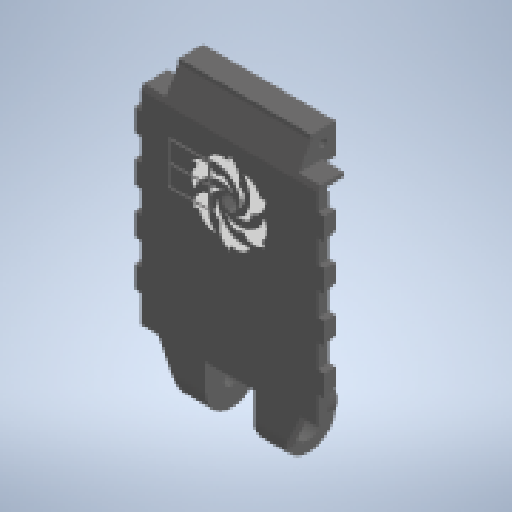
# Autodesk Inventor part: protector
Saved by Autodesk Inventor 2026.1 (Build 301233020, 233B)
## iProperties
Created: 2026-01-21
Part Number: protector
Material: 一般
Document SubType Name: Modeling
Designer: hibik
Density: 1 g/cm^3
Appearance: 既定
Author: hibik
Autodesk Inventor part; units mm, degrees
ref_plane "YZ Plane" through (0, 0, 0) normal (1, 0, 0) x (0, 1, 0)
ref_plane "XZ Plane" through (0, 0, 0) normal (0, 1, 0) x (-1, 0, 0)
ref_plane "XY Plane" through (0, 0, 0) normal (0, 0, 1) x (1, 0, 0)
sketch "スケッチ1" plane through (0, 0, 0) normal (0, 0, 1) x (1, 0, 0)
  line L0 (-20, 22.5) -> (20, 22.5)
  line L1 (20, 22.5) -> (20, -22.5)
  line L2 (20, -22.5) -> (-20, -22.5)
  line L3 (-20, -22.5) -> (-20, 22.5)
  line L4 (-20, 22.5) -> (20, -22.5) construction
  line L5 (20, 22.5) -> (-20, -22.5) construction
  circle A0 centre (-17, 19.5) radius 3
  circle A1 centre (17, -19.5) radius 3
  point P0 (0, 0)
  point P1 (-20, 19.5)
  point P2 (17, -22.5)
  point P3 (20, -19.5)
  point P4 (-17, 22.5)
  dimension "d0" = 40
  dimension "d1" = 45
  dimension "d2" = 6
  constraints: 12 end point, 4 tangent, 2 centre point, 2 midpoint, 2 parallel, 1 equal radius, 1 horizontal, 1 perpendicular
  measures "d0" distance of L0.start L0.end
  measures "d1" distance of L2.end L0.start
  measures "d2" diameter of A0
extrude "押し出し1" add sketch "スケッチ1" along normal blind 0.5 contours L0 L1 A1 L2 L3 A0 | A0 | A1
sketch "スケッチ2" plane through (0, 0, 0) normal (0, 0, -1) x (-1, 0, 0)
  circle A0 centre (17, 19.5) radius 3
  circle A1 centre (-17, -19.5) radius 3
  arc A2 (20, 19.5) -> (17, 22.5) centre (17, 19.5) ccw projected
  arc A3 (-20, -19.5) -> (-17, -22.5) centre (-17, -19.5) ccw projected
  point P0 (0, 0)
  constraints: 4 concentric, 2 centre point
extrude "押し出し2" add sketch "スケッチ2" along normal blind 2
sketch "スケッチ3" plane through (17, -19.5, -2) normal (0, 0, -1) x (-1, 0, 0)
  circle A0 centre (34, 39) radius 1.25
  circle A1 centre (0, 0) radius 1.25
  circle A2 centre (34, 39) radius 3 construction
  circle A3 centre (0, 0) radius 3 construction
  point P0 (17, 19.5)
  dimension "d7" = 2.5
  constraints: 2 centre point, 2 concentric, 1 equal radius
  measures "d7" diameter of A0
extrude "押し出し3" cut sketch "スケッチ3" against normal through all
sketch "スケッチ4" plane through (0, 0, 0.5) normal (0, 0, 1) x (1, 0, 0)
  circle A0 centre (105.92, 111.13) radius 1.6667 projected
  line L0 (-14, 17.5) -> (-4, 17.5)
  line L1 (-4, 17.5) -> (-4, 7.5)
  line L2 (-4, 7.5) -> (-14, 7.5)
  line L3 (-14, 7.5) -> (-14, 17.5)
  line L4 (20, 22.5) -> (-17, 22.5) projected
  line L5 (-20, 19.5) -> (-20, -22.5) projected
  point P0 (0, 0)
  dimension "d10" = 5
  dimension "d11" = 6
  dimension "d12" = 10
  dimension "d13" = 10
  constraints: 8 end point, 2 parallel, 1 horizontal, 1 perpendicular
  measures "d10" distance between parallel lines of L4 L0
  measures "d11" distance between parallel lines of L5 L3
  measures "d12" distance of L0.start L0.end
  measures "d13" distance of L2.end L0.start
extrude "押し出し4" cut sketch "スケッチ4" against normal through all
sketch "スケッチ5" plane through (0, 0, 0.5) normal (0, 0, 1) x (1, 0, 0)
  line L0 (-20, 29.5) -> (20, 29.5)
  line L1 (20, 29.5) -> (20, -22.5)
  line L2 (20, -22.5) -> (-20, -22.5)
  line L3 (-20, -22.5) -> (-20, 29.5)
  line L4 (20, -19.5) -> (20, 22.5) projected
  line L5 (-20, 19.5) -> (-20, -22.5) projected
  line L6 (-20, -22.5) -> (17, -22.5) projected
  line L7 (20, 22.5) -> (-17, 22.5) projected
  line L8 (-14, 17.5) -> (-4, 17.5) projected
  line L9 (-4, 17.5) -> (-4, 7.5) projected
  line L10 (-4, 7.5) -> (-14, 7.5) projected
  line L11 (-14, 7.5) -> (-14, 17.5) projected
  circle A0 centre (0, 11.28) radius 1.6667 projected
  point P0 (0, 0)
  dimension "d16" = 7
  constraints: 8 end point, 3 point on line, 2 parallel, 1 horizontal, 1 perpendicular
  measures "d16" distance between parallel lines of L7 L0
extrude "押し出し5" add sketch "スケッチ5" along normal blind 2
sketch "スケッチ6" plane through (20, -19.5, 0) normal (1, 0, 0) x (0, 0, -1)
  circle A0 centre (3.5, -9) radius 6
  line L0 (-2.5, -3) -> (-2.5, 49) projected
  line L1 (-0.5, -3) -> (-2.5, -3) projected
  line L2 (-0.5, -3) -> (3.5, -3)
  line L3 (-2.5, -3) -> (-2.5, -9)
  point P0 (0, 19.5)
  dimension "d19" = 12
  constraints: 4 end point, 4 tangent, 2 point on circle, 1 centre point
  measures "d19" diameter of A0
extrude "押し出し6" add sketch "スケッチ6" against normal up to surface (40 mm away)
sketch "スケッチ7" plane through (0, 0, 0.5) normal (0, 0, -1) x (-1, 0, 0)
  line L0 (20, 29.5) -> (20, 19.5) projected
  line L1 (-20, 29.5) -> (20, 29.5)
  line L2 (20, 29.5) -> (20, 23.5)
  line L3 (20, 23.5) -> (-20, 23.5)
  line L4 (-20, 23.5) -> (-20, 29.5)
  line L5 (-10, 29.5) -> (10, 29.5)
  line L6 (10, 29.5) -> (10, 23.5)
  line L7 (10, 23.5) -> (-10, 23.5)
  line L8 (-10, 23.5) -> (-10, 29.5)
  line L9 (-20, 22.5) -> (17, 22.5) projected
  line L10 (-11, 29.5) -> (-11, 23.5)
  line L11 (11, 23.5) -> (11, 29.5)
  line L12 (0, 29.5) -> (0, 23.5)
  point P0 (0, 0)
  dimension "d22" = 1
  dimension "d23" = 20
  dimension "d24" = 22
  constraints: 22 end point, 7 point on line, 4 parallel, 4 perpendicular, 3 midpoint, 2 horizontal, 1 other
  measures "d22" distance between parallel lines of L3 L9
  measures "d23" distance between parallel lines of L6 L8
  measures "d24" distance between parallel lines of L10 L11
extrude "押し出し7" cut sketch "スケッチ7" against normal through all contours L0 L3 L11 L1 | L10 L3 L4 L1
extrude "押し出し8" add sketch "スケッチ7" along normal blind 7 contours L11 L3 L6 L1 | L8 L3 L10 L1
extrude "押し出し9" add sketch "スケッチ7" along normal blind 3.5 contours L6 L3 L12 L1 | L12 L3 L8 L1
sketch "スケッチ8" plane through (11, 23.5, 2.5) normal (1, 0, 0) x (0, 0, -1)
  line L0 (0, 0) -> (3.5, 6)
  line L1 (3.5, 6) -> (5.5, 6)
  line L2 (5.5, 6) -> (2, 0)
  line L3 (0, 0) -> (0, 6) projected
  line L4 (0, 6) -> (9, 6) projected
  point P0 (2.5, -23.5)
  constraints: 6 end point, 1 horizontal, 1 parallel
extrude "押し出し10" cut sketch "スケッチ8" against normal through all
sketch "スケッチ9" plane through (0, 0, -6.5) normal (0, 0, -1) x (-1, 0, 0)
  line L0 (-10, 29.5) -> (-11, 29.5) projected
  line L1 (10, 23.5) -> (11, 23.5) projected
  line L2 (-11, 29.5) -> (11, 29.5)
  line L3 (11, 29.5) -> (11, 23.5)
  line L4 (11, 23.5) -> (-11, 23.5)
  line L5 (-11, 23.5) -> (-11, 29.5)
  point P0 (0, 0)
  constraints: 8 end point, 2 parallel, 1 horizontal, 1 perpendicular
extrude "押し出し11" add sketch "スケッチ9" against normal blind 1
sketch "スケッチ10" plane through (-11, 29.5, -6.5) normal (0, 1, 0) x (1, 0, 0)
  line L0 (0, 0) -> (22, 0) projected
  line L1 (0, -5.5) -> (0, 0) projected
  line L2 (0, -5.5) -> (22, -5.5) projected
  line L3 (22, -5.5) -> (22, 0) projected
  line L4 (21, -1) -> (1, -1) projected
  line L5 (21, -3.5) -> (21, -1) projected
  line L6 (1, -3.5) -> (21, -3.5) projected
  line L7 (1, -3.5) -> (1, -1) projected
  point P0 (11, -6.5)
extrude "押し出し12" add sketch "スケッチ10" along normal blind 1 contours L0 L3 L2 L1 | L5 L6 L7 L4
sketch "スケッチ11" plane through (-20, 23.5, 2.5) normal (0, 1, 0) x (1, 0, 0)
  line L0 (9, 0) -> (9, 3.5) projected
  line L1 (31, 3.5) -> (31, 0) projected
  line L2 (31, 3.5) -> (31, 9) projected
  line L3 (9, 9) -> (9, 3.5) projected
  line L4 (0, 0) -> (0, 2) projected
  line L5 (0, 0) -> (9, 0)
  line L6 (9, 0) -> (9, 6)
  line L7 (9, 6) -> (0, 6)
  line L8 (0, 6) -> (0, 0)
  line L9 (40, 0) -> (31, 0)
  line L10 (31, 0) -> (31, 6)
  line L11 (31, 6) -> (40, 6)
  line L12 (40, 6) -> (40, 0)
  point P0 (20, 2.5)
  dimension "d41" = 6
  constraints: 16 end point, 4 parallel, 4 point on line, 2 horizontal, 2 perpendicular
  measures "d41" distance of L7.end L4.start
extrude "押し出し13" add sketch "スケッチ11" along normal blind 1
sketch "スケッチ12" plane through (-20, -22.5, 0) normal (-1, 0, 0) x (0, 0, 1)
  line L0 (1.9167, 47) -> (2.5, 46) projected
  line L1 (2.5, 46) -> (2.5, 47) projected
  line L2 (1.9167, 47) -> (2.5, 47) projected
  point P0 (0, 22.5)
extrude "押し出し14" cut sketch "スケッチ12" against normal through all
sketch "スケッチ13" plane through (0, 0, 0) normal (1, 0, 0) x (0, 1, 0)
  line L0 (24.5, 1.9167) -> (23.5, 2.5) projected
  line L1 (23.5, 2.5) -> (-28.5, 2.5) projected
  arc A0 (-28.5, 2.5) -> (-22.5, -3.5) centre (-28.5, -3.5) ccw projected
  line L2 (-22.5, -3.5) -> (-22.5, 0.5) projected
  line L3 (-22.5, 0.5) -> (-19.5, 0.5) projected
  line L4 (-19.5, 0) -> (-19.5, 0.5) projected
  line L5 (-19.5, 0) -> (22.5, 0) projected
  line L6 (22.5, 0) -> (22.5, 0.5) projected
  line L7 (22.5, 0.5) -> (23.5, 0.5) projected
  line L8 (23.5, 0.5) -> (23.5, -3.5) projected
  line L9 (23.5, -3.5) -> (24.5, -3.5) projected
  line L10 (24.5, 1.9167) -> (24.5, -3.5) projected
  line L11 (-22.5, 0.5) -> (-22.5, 2.5)
  point P0 (0, 0)
  constraints: 2 end point, 1 perpendicular, 1 point on line
extrude "押し出し15" cut sketch "スケッチ13" along normal mid plane 11 contours L11 L2 A0 L1
sketch "スケッチ14" plane through (20, -19.5, 0) normal (1, 0, 0) x (0, 0, -1)
  line L0 (-1.9167, 44) -> (-2.5, 43) projected
  line L1 (-2.5, 43) -> (-2.5, -9) projected
  arc A0 (-2.5, -9) -> (3.5, -3) centre (3.5, -9) ccw projected
  line L2 (3.5, -3) -> (-0.5, -3) projected
  line L3 (-0.5, -3) -> (-0.5, 0) projected
  line L4 (0, 0) -> (-0.5, 0) projected
  line L5 (0, 0) -> (0, 42) projected
  line L6 (0, 42) -> (-0.5, 42) projected
  line L7 (-0.5, 42) -> (-0.5, 43) projected
  line L8 (-0.5, 43) -> (3.5, 43) projected
  line L9 (3.5, 43) -> (3.5, 44) projected
  line L10 (-1.9167, 44) -> (3.5, 44) projected
  line L11 (-0.5, -3) -> (-2.5, -3)
  point P0 (0, 19.5)
  constraints: 2 end point, 1 perpendicular, 1 point on line
extrude "押し出し16" cut sketch "スケッチ14" against normal blind 8 contours L11 L2 A0 L1
chamfer "面取り3" distance 4 distance2 9 2 edges at (12, -22.5, 1.5) (12, -22.5, 0.25) measured on face at (12.5, -22.5, 0.25) measured on face at (12.5, -22.5, 1.5)
sketch "スケッチ15" plane through (12, -19.5, 0) normal (1, 0, 0) x (0, 0, -1)
  line L0 (-1.6962, -12) -> (0, -12) projected
  arc A0 (-1.6962, -12) -> (3.5, -3) centre (3.5, -9) ccw projected
  line L1 (0, -3) -> (3.5, -3) projected
  line L2 (0, -3) -> (0, -12) projected
  circle A1 centre (3.5, -9) radius 1.75
  point P0 (0, 19.5)
  dimension "d56" = 3.5
  constraints: 1 centre point, 1 coincident
  measures "d56" diameter of A1
extrude "押し出し17" cut sketch "スケッチ15" against normal through all contours A1
mirror "ミラー1" about plane through (0, 0, 0) normal (1, 0, 0) of "押し出し16", "面取り3"
sketch "スケッチ16" plane through (12, -19.5, 0) normal (1, 0, 0) x (0, 0, -1)
  circle A0 centre (3.5, -9) radius 1.75 projected
  circle A1 centre (3.5, -9) radius 3.5
  point P0 (0, 19.5)
  dimension "d59" = 7
  constraints: 1 centre point, 1 coincident
  measures "d59" diameter of A1
extrude "押し出し18" cut sketch "スケッチ16" against normal blind 3
sketch "スケッチ17" plane through (-12, -31.5, 0) normal (-1, 0, 0) x (0, 0, 1)
  circle A0 centre (-3.5, 3) radius 1.75 projected
  arc A1 (-3.5, 9) -> (2.5, 3) centre (-3.5, 3) ccw projected
  line L0 (-3.5, -1.0415) -> (-7, 0.9793)
  line L1 (-7, 0.9793) -> (-7, 5.0207)
  line L2 (-7, 5.0207) -> (-3.5, 7.0415)
  line L3 (-3.5, 7.0415) -> (0, 5.0207)
  line L4 (0, 5.0207) -> (0, 0.9793)
  line L5 (0, 0.9793) -> (-3.5, -1.0415)
  point P0 (0, 31.5)
  dimension "d62" = 7
  constraints: 12 end point, 1 coincident, 1 vertical, 13 other
  measures "d62" distance between parallel lines of L4 L1
extrude "押し出し19" cut sketch "スケッチ17" against normal blind 3
sketch "スケッチ18" plane through (0, 0, 0) normal (0, 0, -1) x (-1, 0, 0)
  line L0 (4, 12.75) -> (13.5, 12.75)
  line L1 (13.5, 12.75) -> (13.5, 17)
  line L2 (13.5, 17) -> (4, 17)
  line L3 (4, 17) -> (4, 12.75)
  line L4 (4, 12.25) -> (13.5, 12.25)
  line L5 (13.5, 12.25) -> (13.5, 8)
  line L6 (13.5, 8) -> (4, 8)
  line L7 (4, 8) -> (4, 12.25)
  line L8 (4, 7.5) -> (4, 17.5) projected
  line L9 (14, 17.5) -> (14, 7.5) projected
  line L10 (4, 17.5) -> (14, 17.5) projected
  line L11 (14, 7.5) -> (4, 7.5) projected
  point P0 (0, 0)
  dimension "d65" = 0.5
  dimension "d66" = 0.5
  dimension "d67" = 0.5
  dimension "d68" = 0.5
  constraints: 16 end point, 4 parallel, 3 collinear, 2 horizontal, 2 perpendicular, 1 point on line
  measures "d65" distance between parallel lines of L9 L5
  measures "d66" distance between parallel lines of L0 L4
  measures "d67" distance between parallel lines of L10 L2
  measures "d68" distance between parallel lines of L11 L6
extrude "押し出し20" add sketch "スケッチ18" against normal blind 1 contours L3 L2 L1 L0 | L4 L5 L6 L7
sketch "スケッチ19" plane through (0, 0, 1) normal (0, 0, 1) x (1, 0, 0)
  line L0 (-4, 17) -> (-13.5, 17) projected
  line L1 (-13.5, 17) -> (-13.5, 12.75) projected
  line L2 (-13.5, 12.75) -> (-4, 12.75) projected
  line L3 (-4, 17) -> (-4, 12.75) projected
  line L4 (-4, 12.25) -> (-13.5, 12.25) projected
  line L5 (-13.5, 12.25) -> (-13.5, 8) projected
  line L6 (-13.5, 8) -> (-4, 8) projected
  line L7 (-4, 12.25) -> (-4, 8) projected
  line L8 (-13.5, 17) -> (-4, 17) projected
  line L9 (-5, 17) -> (-4, 17)
  line L10 (-4, 17) -> (-4, 8)
  line L11 (-4, 8) -> (-5, 8)
  line L12 (-5, 8) -> (-5, 17)
  point P0 (0, 0)
  point P1 (-5, 12.25)
  point P2 (-5, 12.75)
  dimension "d71" = 1
  constraints: 8 end point, 2 parallel, 1 horizontal, 1 perpendicular, 1 point on line
  measures "d71" distance between parallel lines of L3 L12
extrude "押し出し21" add sketch "スケッチ19" along normal blind 1.5 contours L12 L2 L1 L0 | L12 L6 L5 L4
sketch "スケッチ22" plane through (0, 0, 2.5) normal (0, 0, 1) x (1, 0, 0)
  arc A0 (2.3857, 13.635) -> (-4.7391, 17.5727) centre (-3.1979, 11.9467) ccw projected
  arc A1 (2.3333, 11.5467) -> (2.3857, 13.635) centre (-0.8049, 12.6703) ccw projected
  arc A2 (2.3333, 11.5467) -> (3.2246, 14.6133) centre (-2.442, 14.5974) ccw projected
  arc A3 (3.2246, 14.6133) -> (2.091, 15.8291) centre (0.9333, 13.6133) ccw projected
  arc A4 (2.091, 15.8291) -> (-0.4466, 20.7823) centre (-1.7789, 16.9731) ccw projected
  arc A5 (-0.8333, 19.5075) -> (-0.4466, 20.7823) centre (-0.6667, 20.153) ccw projected
  arc A6 (-0.8333, 19.5075) -> (-4.7391, 17.5727) centre (-1.6667, 16.28) ccw projected
  arc A7 (3.2324, 10.3914) -> (3.0801, 18.5306) centre (-1.0216, 14.3828) ccw projected
  arc A8 (1.3976, 9.3926) -> (3.2324, 10.3914) centre (0.8015, 12.6722) ccw projected
  arc A9 (1.3976, 9.3926) -> (4.4991, 10.1541) centre (1.652, 15.0536) ccw projected
  arc A10 (4.4991, 10.1541) -> (4.9852, 11.7437) centre (2.4874, 11.6384) ccw projected
  arc A11 (4.9852, 11.7437) -> (8.0059, 16.4179) centre (4.0409, 15.6671) ccw projected
  arc A12 (6.7085, 16.1154) -> (8.0059, 16.4179) centre (7.3509, 16.2938) ccw projected
  arc A13 (6.7085, 16.1154) -> (3.0801, 18.5306) centre (3.4968, 15.2234) ccw projected
  arc A14 (-0.8467, 14.5236) -> (-7.8192, 10.3222) centre (-2.1763, 8.8439) ccw projected
  arc A15 (0.9357, 13.4341) -> (-0.8467, 14.5236) centre (-1.6065, 11.278) ccw projected
  arc A16 (0.9357, 13.4341) -> (-1.2744, 15.7393) centre (-4.094, 10.8239) ccw projected
  arc A17 (-1.2744, 15.7393) -> (-2.8942, 15.3654) centre (-1.5541, 13.255) ccw projected
  arc A18 (-2.8942, 15.3654) -> (-8.4525, 15.6444) centre (-5.8198, 12.586) ccw projected
  arc A19 (-7.5419, 14.6721) -> (-8.4525, 15.6444) centre (-8.0176, 15.1391) ccw projected
  arc A20 (-7.5419, 14.6721) -> (-7.8192, 10.3222) centre (-5.1635, 12.3366) ccw projected
  arc A21 (-3.2324, 12.1686) -> (-3.0801, 4.0294) centre (1.0216, 8.1772) ccw projected
  arc A22 (-1.3976, 13.1674) -> (-3.2324, 12.1686) centre (-0.8015, 9.8878) ccw projected
  arc A23 (-1.3976, 13.1674) -> (-4.4991, 12.4059) centre (-1.652, 7.5064) ccw projected
  arc A24 (-4.4991, 12.4059) -> (-4.9852, 10.8163) centre (-2.4874, 10.9216) ccw projected
  arc A25 (-4.9852, 10.8163) -> (-8.0059, 6.1421) centre (-4.0409, 6.8929) ccw projected
  arc A26 (-6.7085, 6.4446) -> (-8.0059, 6.1421) centre (-7.3509, 6.2662) ccw projected
  arc A27 (-6.7085, 6.4446) -> (-3.0801, 4.0294) centre (-3.4968, 7.3366) ccw projected
  arc A28 (-2.3857, 8.925) -> (4.7391, 4.9873) centre (3.1979, 10.6133) ccw projected
  arc A29 (-2.3333, 11.0133) -> (-2.3857, 8.925) centre (0.8049, 9.8897) ccw projected
  arc A30 (-2.3333, 11.0133) -> (-3.2246, 7.9467) centre (2.442, 7.9626) ccw projected
  arc A31 (-3.2246, 7.9467) -> (-2.091, 6.7309) centre (-0.9333, 8.9467) ccw projected
  arc A32 (-2.091, 6.7309) -> (0.4466, 1.7777) centre (1.7789, 5.5869) ccw projected
  arc A33 (0.8333, 3.0525) -> (0.4466, 1.7777) centre (0.6667, 2.407) ccw projected
  arc A34 (0.8333, 3.0525) -> (4.7391, 4.9873) centre (1.6667, 6.28) ccw projected
  arc A35 (0.8467, 8.0364) -> (7.8192, 12.2378) centre (2.1763, 13.7161) ccw projected
  arc A36 (-0.9357, 9.1259) -> (0.8467, 8.0364) centre (1.6065, 11.282) ccw projected
  arc A37 (-0.9357, 9.1259) -> (1.2744, 6.8207) centre (4.094, 11.7361) ccw projected
  arc A38 (1.2744, 6.8207) -> (2.8942, 7.1946) centre (1.5541, 9.305) ccw projected
  arc A39 (2.8942, 7.1946) -> (8.4525, 6.9156) centre (5.8198, 9.974) ccw projected
  arc A40 (7.5419, 7.8879) -> (8.4525, 6.9156) centre (8.0176, 7.4209) ccw projected
  arc A41 (7.5419, 7.8879) -> (7.8192, 12.2378) centre (5.1635, 10.2234) ccw projected
  point P0 (0, 0)
extrude "押し出し22" cut sketch "スケッチ22" against normal blind 0.01
sketch "スケッチ28" plane through (0, 0, 2.5) normal (0, 0, 1) x (1, 0, 0)
  arc A0 (-2.8942, 15.3654) -> (-8.4525, 15.6444) centre (-5.8198, 12.586) ccw projected
  arc A1 (-7.5419, 14.6721) -> (-8.4525, 15.6444) centre (-8.0176, 15.1391) ccw projected
  arc A2 (-7.5419, 14.6721) -> (-7.8192, 10.3222) centre (-5.1635, 12.3366) ccw projected
  arc A3 (-0.8467, 14.5236) -> (-7.8192, 10.3222) centre (-2.1763, 8.8439) ccw projected
  arc A4 (-4.9852, 10.8163) -> (-8.0059, 6.1421) centre (-4.0409, 6.8929) ccw projected
  line L0 (-13.5, 8) -> (-5, 8) projected
  line L1 (-5, 8) -> (-5, 12.25) projected
  line L2 (-13.5, 12.75) -> (-5, 12.75) projected
  line L3 (-5, 12.75) -> (-5, 17) projected
  point P0 (0, 0)
  point P1 (-5, 10.8127)
  point P2 (-7.9215, 8)
  point P3 (-8.4711, 12.75)
  point P4 (-6.5087, 12.75)
  point P5 (-5, 13.9482)
  point P6 (-5, 16.5373)
extrude "押し出し28" cut sketch "スケッチ28" against normal blind 0.01 contours L3 A3 L2 A2 A1 A0 | A3 A2 L2 | L1 L0 A4
sketch "スケッチ29" plane through (0, 0, 1) normal (0, 0, 1) x (1, 0, 0)
  line L0 (-5, 17) -> (-5, 12.75) projected
  line L1 (-5, 12.75) -> (-4, 12.75) projected
  line L2 (-4, 17) -> (-4, 12.75) projected
  line L3 (-4, 17) -> (-5, 17) projected
  line L4 (-5, 12.25) -> (-5, 8) projected
  line L5 (-5, 8) -> (-4, 8) projected
  line L6 (-4, 12.25) -> (-4, 8) projected
  line L7 (-4, 12.25) -> (-5, 12.25) projected
  arc A0 (-4.4991, 12.4059) -> (-4.9852, 10.8163) centre (-2.4874, 10.9216) ccw projected
  arc A1 (-3.2324, 12.1686) -> (-3.0801, 4.0294) centre (1.0216, 8.1772) ccw projected
  arc A2 (-0.8467, 14.5236) -> (-7.8192, 10.3222) centre (-2.1763, 8.8439) ccw projected
  arc A3 (-2.8942, 15.3654) -> (-8.4525, 15.6444) centre (-5.8198, 12.586) ccw projected
  arc A4 (-4.9852, 10.8163) -> (-8.0059, 6.1421) centre (-4.0409, 6.8929) ccw projected
  point P0 (0, 0)
  point P1 (-5, 10.8127)
  point P2 (-4.809, 8)
  point P3 (-4, 11.1456)
  point P4 (-4.6053, 12.25)
  point P5 (-4, 16.1878)
  point P6 (-5, 16.5373)
  point P7 (-5, 13.9482)
  point P8 (-4, 14.3848)
extrude "押し出し29" cut sketch "スケッチ29" against normal blind 0.01 contours A3 L2 A2 L0 | A4 A0 L7 L6 A1 L5 L4
sketch "スケッチ30" plane through (0, 0, 2.5) normal (0, 0, 1) x (1, 0, 0)
  line L0 (20, -19.5) -> (20, 22.5) projected
  line L1 (20, 19.5) -> (21.5, 19.5)
  line L2 (21.5, 19.5) -> (21.5, 14.5)
  line L3 (21.5, 14.5) -> (20, 14.5)
  line L4 (20, 14.5) -> (20, 19.5)
  line L5 (11, 24.5) -> (20, 24.5) projected
  line L6 (20, 9.25) -> (21.5, 9.25)
  line L7 (21.5, 9.25) -> (21.5, 4.25)
  line L8 (21.5, 4.25) -> (20, 4.25)
  line L9 (20, -1) -> (21.5, -1)
  line L10 (21.5, -1) -> (21.5, -6)
  line L11 (21.5, -6) -> (20, -6)
  line L12 (20, -11.25) -> (21.5, -11.25)
  line L13 (21.5, -11.25) -> (21.5, -16.25)
  line L14 (21.5, -16.25) -> (20, -16.25)
  point P0 (0, 0)
  dimension "d92" = 1.5
  dimension "d93" = 5
  dimension "d94" = 5
  dimension "d97" = 10.25
  constraints: 26 end point, 2 parallel, 1 horizontal, 1 perpendicular, 1 point on line, 1 vertical, 21 other
  measures "d92" distance of L2.end L3.end
  measures "d93" distance of L1.end L2.end
  measures "d94" distance between parallel lines of L5 L1
  measures "d97" distance of L1.start L6.start
extrude "押し出し30" add sketch "スケッチ30" against normal up to surface (2.5 mm away)
chamfer "面取り4" distance 1 distance2 2.5 4 edges at (20.75, 14.5, 0) (20.75, 4.25, 0) (20.75, -6, 0) (20.75, -16.25, 0)
mirror "ミラー2" about plane through (0, 0, 0) normal (1, 0, 0) of "押し出し30", "面取り4"
sketch "スケッチ32" plane through (0, 11.28, 0.5) normal (0, 0, 1) x (1, 0, 0)
  circle A0 centre (0, 0) radius 1.6667 projected
  point P0 (0, -11.28)
extrude "押し出し32" cut sketch "スケッチ32" against normal through all
sketch "スケッチ33" plane through (0, 0, 0) normal (0, 0, -1) x (-1, 0, 0)
  line L0 (5, 16.5373) -> (5, 17) projected
  line L1 (5, 17) -> (13.5, 17) projected
  line L2 (13.5, 17) -> (13.5, 12.75) projected
  line L3 (13.5, 12.75) -> (8.4711, 12.75) projected
  line L4 (6, 17) -> (13.5, 17)
  line L5 (13.5, 17) -> (13.5, 12.75)
  line L6 (13.5, 12.75) -> (6, 12.75)
  line L7 (6, 12.75) -> (6, 17)
  line L8 (6, 12.25) -> (13.5, 12.25)
  line L9 (13.5, 12.25) -> (13.5, 8)
  line L10 (13.5, 8) -> (6, 8)
  line L11 (6, 8) -> (6, 12.25)
  line L12 (13.5, 12.25) -> (4, 12.25) projected
  line L13 (4, 8) -> (13.5, 8) projected
  point P0 (0, 0)
  dimension "d112" = 1
  constraints: 16 end point, 4 parallel, 3 point on line, 2 collinear, 2 horizontal, 2 perpendicular
  measures "d112" distance from line of L7 L0.start
extrude "押し出し33" cut sketch "スケッチ33" against normal blind 1
fillet "フィレット2" radius 1 2 edges at (-6, 14.875, 1) (-6, 10.125, 1)
sketch "スケッチ34" plane through (0, 0, 0) normal (0, 0, -1) x (-1, 0, 0)
  line L0 (-19, 14.5) -> (-6, 14.5)
  line L1 (-6, 14.5) -> (-6, -5.5)
  line L2 (-6, -5.5) -> (-19, -5.5)
  line L3 (-19, -5.5) -> (-19, 14.5)
  line L4 (-20, 9.25) -> (-20, 15.5) projected
  line L5 (20, 23.5) -> (-20, 23.5) projected
  point P0 (0, 0)
  dimension "d116" = 1
  dimension "d117" = 9
  dimension "d118" = 20
  dimension "d119" = 13
  constraints: 8 end point, 2 parallel, 1 horizontal, 1 perpendicular
  measures "d116" distance between parallel lines of L4 L3
  measures "d117" distance between parallel lines of L5 L0
  measures "d118" distance of L2.end L0.start
  measures "d119" distance of L0.start L0.end
extrude "押し出し34" cut sketch "スケッチ34" against normal blind 2
sketch "スケッチ35" plane through (11, 23.5, -6.5) normal (1, 0, 0) x (0, 0, -1)
  line L0 (-8.4167, 1) -> (-3, 1) projected
  line L1 (-3, 1) -> (-3, 0) projected
  line L2 (-3, 0) -> (0, 0) projected
  line L3 (0, 0) -> (0, 7) projected
  line L4 (-5.5, 7) -> (0, 7) projected
  line L5 (-5.5, 6) -> (-5.5, 7) projected
  line L6 (-5.5, 6) -> (-8.4167, 1) projected
  circle A0 centre (-2.75, 4) radius 0.8
  line L7 (-5.5, 7) -> (0, 7) projected
  point P0 (-6.5, -23.5)
  point P1 (-2.75, 7)
  dimension "d122" = 1.6
  dimension "d123" = 3
  constraints: 1 centre point, 1 midpoint, 1 vertical alignment
  measures "d122" diameter of A0
  measures "d123" distance from line of L4 A0.centre
extrude "押し出し35" add sketch "スケッチ35" along normal blind 4
mirror "ミラー3" about plane through (0, 0, 0) normal (1, 0, 0) of "押し出し35"
